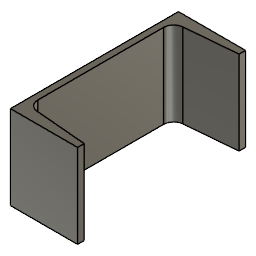
C-200×80×7.5×11 (Autodesk Fusion 360 design; units mm, degrees)
Autodesk Fusion 360 part; units mm, degrees
sketch "スケッチ1" plane through (0, 0, 0) normal (0, 0, 1) x (1, 0, 0)
  line L0 (7.5, 174.8326) -> (7.5, 25.1674)
  line L1 (0, 200) -> (0, 0)
  line L2 (0, 0) -> (80, 0)
  line L3 (80, 7.8285) -> (80, 0)
  line L4 (18.4541, 13.2131) -> (80, 7.8285)
  arc A0 (7.5, 25.1674) -> (18.4541, 13.2131) centre (19.5, 25.1674) ccw
  line L5 (80, 192.1715) -> (18.4541, 186.7869)
  line L6 (0, 200) -> (80, 200)
  arc A1 (18.4541, 186.7869) -> (7.5, 174.8326) centre (19.5, 174.8326) ccw
  line L7 (80, 200) -> (80, 192.1715)
extrude "押し出し1" add sketch "スケッチ1" along normal blind 100
